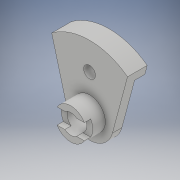
# Autodesk Inventor part: C
Saved by Autodesk Inventor 2018 (Build 220112000, 112)
## iProperties
Created: 2017-09-30
Part Number: C
Material: Generic
Document SubType Name: Modeling
Designer: Soichi
Density: 1 g/cm^3
Appearance: Default
Author: Soichi
Autodesk Inventor part; units mm, degrees
ref_plane "YZ Plane" through (0, 0, 0) normal (1, 0, 0) x (0, 1, 0)
ref_plane "XZ Plane" through (0, 0, 0) normal (0, 1, 0) x (-1, 0, 0)
ref_plane "XY Plane" through (0, 0, 0) normal (0, 0, 1) x (1, 0, 0)
sketch "Sketch1" plane through (0, 0, 0) normal (0, 1, 0) x (-1, 0, 0)
  circle A0 centre (0, 0) radius 30
  circle A1 centre (0, 0) radius 20
  circle A2 centre (0, 0) radius 12.5
  line L0 (0, 0) -> (0, -45) construction
  circle A3 centre (0, -45) radius 7.5
  line L1 (-21, 10) -> (21, 10)
  line L2 (21, 10) -> (21, -10)
  line L3 (21, -10) -> (-21, -10)
  line L4 (-21, -10) -> (-21, 10)
  line L5 (-21, 10) -> (21, -10) construction
  line L6 (21, 10) -> (-21, -10) construction
  line L7 (28.9778, 7.7646) -> (48.1723, -63.8704)
  line L8 (-28.9778, 7.7646) -> (-48.1723, -63.8704)
  arc A4 (-48.1723, -63.8704) -> (48.1723, -63.8704) centre (0, 0) ccw
  arc A5 (-45.129, -52.5126) -> (45.129, -52.5126) centre (0, 0) ccw
  dimension "d0" = 60
  dimension "d1" = 40
  dimension "d2" = 25
  dimension "d5" = 45
  dimension "d6" = 15
  dimension "d7" = 42
  dimension "d8" = 20
  dimension "d11" = 80
  dimension "d12" = 30
  dimension "d13" = 15
  dimension "d19" = 69.2401
  constraints: 18 end point, 7 coincident, 6 centre point, 6 point on circle, 2 midpoint, 2 parallel, 2 point on line, 2 tangent, 1 horizontal, 1 perpendicular, 1 vertical
  measures "d0" diameter of A0
  measures "d1" diameter of A1
  measures "d2" diameter of A2
  measures "d5" distance of L0.start L0.end
  measures "d6" diameter of A3
  measures "d7" distance of L2.end L3.end
  measures "d8" distance of L1.end L2.end
  measures "d11" radius of A4
  measures "d12" angle of L7 L8
  measures "d13" angle of L0 L8
  measures "d19" radius of A5
extrude "Extrusion1" add sketch "Sketch1" along normal blind 24 contours A1 L3 A2 L1 | L1 A2 A1 | A1 L3 A2 | L1 A2 L3 A1
extrude "Extrusion2" cut sketch "Sketch1" against normal blind 8 from surface at 24 contours A0 | A1 L3 A2 L1 | A1 L1 L2 L3 | L1 A2 L3 A1 | A1 L3 L4 L1 | A2 L3 L1
extrude "Extrusion3" add sketch "Sketch1" against normal blind 25 contours L7 A4 L8 A5
extrude "Extrusion4" add sketch "Sketch1" against normal blind 12 contours A0 | A0 L7 A5 L8 | A1 L3 A2 L1 | A1 L1 L2 L3 | L1 A2 A1 | A1 L3 A2 | L1 A2 L3 A1 | A1 L3 L4 L1 | L1 A2 | A2 L3 L1 | A2 L3
body "Solid1"
